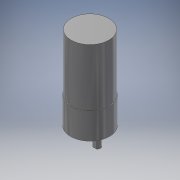
# Autodesk Inventor part: rs380ph_36
Saved by Autodesk Inventor 2017 (Build 210142000, 142)
## iProperties
Created: 2011-03-04
Part Number: rs380ph_36
Document SubType Name: Modeling
Designer: Seiji
Density: 3.94315 g/cm^3
Mass: 270 g
Surface Area: 102.094 cm^2
Volume: 68.4732 cm^3
Material: Steel
Appearance: 鋼
Author: Seiji
Autodesk Inventor part; units mm, degrees
ref_plane "YZ Plane" through (0, 0, 0) normal (1, 0, 0) x (0, 1, 0)
ref_plane "XZ Plane" through (0, 0, 0) normal (0, 1, 0) x (-1, 0, 0)
sketch "スケッチ1" plane through (0, 0, 0) normal (0, 0, 1) x (1, 0, 0)
  circle A0 centre (0, 0) radius 18.5
  dimension "d0" = 37
  constraints: 1 centre point
  measures "d0" diameter of A0
extrude "押し出し1" add sketch "スケッチ1" along normal blind 25
sketch "スケッチ2" plane through (0, 0, 25) normal (0, 0, 1) x (1, 0, 0)
  circle A0 centre (0, 0) radius 18
  dimension "d3" = 36
  constraints: 1 centre point
  measures "d3" diameter of A0
extrude "押し出し2" add sketch "スケッチ2" along normal blind 54.5
sketch "スケッチ3" plane through (0, 0, 0) normal (0, 0, -1) x (-1, 0, 0)
  circle A0 centre (0, 0) radius 18.5 projected
  circle A1 centre (0, 7) radius 6
  dimension "d6" = 12
  dimension "d7" = 7
  constraints: 1 centre point, 1 vertical alignment
  measures "d6" diameter of A1
  measures "d7" distance of A0.centre A1.centre
extrude "押し出し3" add sketch "スケッチ3" along normal blind 6 contours A1
sketch "スケッチ4" plane through (0, 7, -6) normal (0, 0, -1) x (-1, 0, 0)
  circle A0 centre (0, 0) radius 3
  point P0 (0, -7)
  dimension "d10" = 6
  constraints: 1 centre point
  measures "d10" diameter of A0
extrude "押し出し4" add sketch "スケッチ4" along normal blind 15
sketch "スケッチ5" plane through (0, 0, 0) normal (0, 0, -1) x (-1, 0, 0)
  circle A0 centre (0, 0) radius 18.5 projected
  circle A1 centre (0, 0) radius 15.5
  line L0 (0, 0) -> (-15.5, 0)
  line L1 (7.75, 13.4234) -> (0, 0)
  line L2 (0, 0) -> (7.75, -13.4234)
  point P0 (-15.5, 0)
  point P1 (7.75, -13.4234)
  dimension "d13" = 31
  dimension "d14" = 120
  dimension "d15" = 120
  constraints: 6 end point, 5 coincident, 3 point on circle, 1 centre point, 1 horizontal
  measures "d13" diameter of A1
  measures "d14" angle of L2 L0
  measures "d15" angle of L1 L2
hole "Hole1" at (15.5, 0, 0) at (-7.75, -13.4234, 0) at (-7.75, 13.4234, 0) direction (0, 0, 1) diameter 3 depth 3 tip angle 118
ref_plane "作業平面1" through (0, 0, 0) normal (1, 0, 0) x (0, 0.3162, -0.9487)
sketch "スケッチ7" plane through (0, 7, -21) normal (0, 0, -1) x (-1, 0, 0)
  line L0 (1.6583, -2.5) -> (-1.6583, -2.5)
  circle A0 centre (0, 0) radius 3 projected
  point P0 (0, -7)
  dimension "d33" = 2.5
  constraints: 2 end point, 2 point on circle, 1 horizontal
  measures "d33" distance from line of A0.centre L0
extrude "押し出し5" cut sketch "スケッチ7" against normal blind 12 contours A0 L0 picked at (0.3442, -2.6056)
